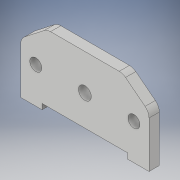
# Autodesk Inventor part: Tope riel final
Saved by Autodesk Inventor 2019 (Build 230136000, 136)
## iProperties
Created: 2020-02-01
Part Number: Tope riel final
Material: Generic
Document SubType Name: Modeling
Designer: Elías Sánchez
Density: 1 g/cm^3
Appearance: Default
Author: Elías Sánchez
Autodesk Inventor part; units mm, degrees
ref_plane "YZ Plane" through (0, 0, 0) normal (1, 0, 0) x (0, 1, 0)
ref_plane "XZ Plane" through (0, 0, 0) normal (0, 1, 0) x (-1, 0, 0)
ref_plane "XY Plane" through (0, 0, 0) normal (0, 0, 1) x (1, 0, 0)
sketch "Sketch1" plane through (0, 0, 0) normal (0, 0, 1) x (1, 0, 0)
  line L0 (37.5, 0) -> (37.5, 30)
  line L1 (37.5, 30) -> (22.1407, 42)
  line L2 (22.1407, 42) -> (-22.1407, 42)
  line L3 (-22.1407, 42) -> (-37.5, 30)
  line L4 (-37.5, 30) -> (-37.5, 0)
  circle A0 centre (-28.678, 21) radius 3.5
  circle A1 centre (28.678, 21) radius 3.5
  circle A2 centre (0, 21) radius 3.75
  line L5 (-37.5, 0) -> (-25, 0)
  line L6 (-25, 0) -> (-25, 3.2)
  line L7 (-25, 3.2) -> (25, 3.2)
  line L8 (25, 3.2) -> (25, 0)
  line L9 (25, 0) -> (37.5, 0)
  line L10 (0, -8.4) -> (0, 50.4) projected
  line L11 (-52.5, 0) -> (52.5, 0) projected
  point P0 (0, 0)
  point P1 (0, 42)
  point P2 (0, 0)
  dimension "d0" = 30
  dimension "d1" = 30
  dimension "d3" = 128
  dimension "d4" = 75
  dimension "d5" = 7
  dimension "d7" = 7
  dimension "d9" = 28.678
  dimension "d10" = 28.678
  dimension "d24" = 7.5
  dimension "d28" = 50
  dimension "d29" = 12.5
  dimension "d30" = 3.2
  dimension "d31" = 37.5
  dimension "d32" = 128
  dimension "d33" = 3.2
  dimension "d34" = 17.8
  dimension "d36" = 44.2814
  constraints: 20 end point, 4 perpendicular, 3 centre point, 2 coincident, 2 horizontal alignment, 2 vertical alignment, 1 horizontal, 1 midpoint, 1 parallel, 1 point on line
  measures "d0" distance of L3.end L4.end
  measures "d1" distance of L0.start L0.end
  measures "d3" angle of L0 L1
  measures "d4" distance of L4.end L0.start
  measures "d5" diameter of A0
  measures "d7" diameter of A1
  measures "d9" horizontal distance of point (0, 0) A1.centre
  measures "d10" horizontal distance of point (0, 0) A0.centre
  measures "d24" diameter of A2
  measures "d28" distance of L6.end L7.end
  measures "d29" distance of L4.end L5.end
  measures "d30" distance between parallel lines of L9 L7
  measures "d31" distance between parallel lines of L10 L0
  measures "d32" angle of L4 L3
  measures "d33" distance between parallel lines of L7 L11
  measures "d34" distance from line of L7 A2.centre
  measures "d36" distance of L1.end L2.end
extrude "Extrusion2" add sketch "Sketch1" along normal blind 6 contours L9 L8 L7 L10 A2 L2 L1 L0 | L10 A2 L7 L6 L5 L4 L3 L2
fillet "Fillet2" radius 6 4 edges at (-22.1407, 42, 3) (22.1407, 42, 3) (37.5, 30, 3) (-37.5, 30, 3)
equation "\"d1\" = d0"
equation "\"d7\" = d5"
equation "\"d10\" = d9"
body "Solid2"
